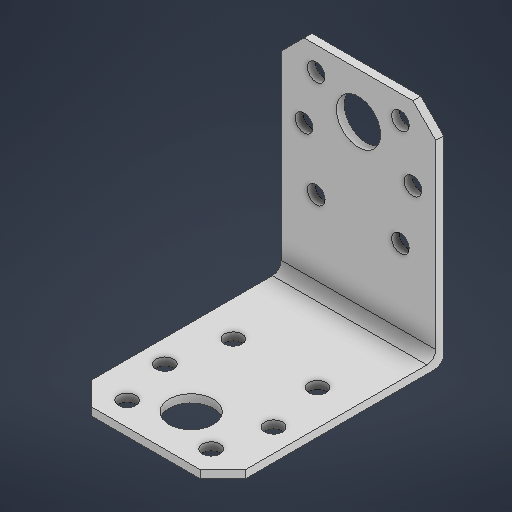
# Autodesk Inventor part: угол для катушки
Saved by Autodesk Inventor 2025 (Build 290162000, 162)
## iProperties
Created: 2025-01-08
Part Number: угол для катушки
Material: Типовые
Document SubType Name: Modeling
Designer: GameHD
Density: 1 g/cm^3
Appearance: По умолчанию
Author: GameHD
Autodesk Inventor part; units mm, degrees
ref_plane "YZ Plane" through (0, 0, 0) normal (1, 0, 0) x (0, 1, 0)
ref_plane "XZ Plane" through (0, 0, 0) normal (0, 1, 0) x (-1, 0, 0)
ref_plane "XY Plane" through (0, 0, 0) normal (0, 0, 1) x (1, 0, 0)
sketch "Эскиз1" plane through (0, 0, 0) normal (0, 0, 1) x (1, 0, 0)
  line L0 (0, 0) -> (35, 0)
  line L1 (35, 0) -> (35, 50)
  line L2 (35, 50) -> (0, 50)
  line L3 (0, 50) -> (0, 0)
  dimension "d0" = 35
  dimension "d1" = 50
  constraints: 8 end point, 2 parallel, 1 horizontal, 1 perpendicular
  measures "d0" distance of L2.end L1.end
  measures "d1" distance of L1.end L0.end
extrude "Выдавливание1" add sketch "Эскиз1" along normal blind 1.8
sketch "Эскиз2" plane through (0, 0, 1.8) normal (0, 0, 1) x (1, 0, 0)
  line L0 (0, 0) -> (35, 0)
  line L1 (35, 0) -> (35, 1.8)
  line L2 (35, 1.8) -> (0, 1.8)
  line L3 (0, 1.8) -> (0, 0)
  dimension "d5" = 35
  dimension "d6" = 1.8
  constraints: 8 end point, 2 parallel, 1 horizontal, 1 perpendicular
  measures "d5" distance of L2.end L1.end
  measures "d6" distance of L1.end L0.end
extrude "Выдавливание2" add sketch "Эскиз2" along normal blind 48.2
fillet "Сопряжение1" radius 2 2 edges at (17.5, 1.8, 1.8) (17.5, 0, 0)
chamfer "Фаска1" distance 5.175 angle 45 4 edges at (0, 50, 0.9) (0, 0.9, 50) (35, 0.9, 50) (35, 50, 0.9)
sketch "Эскиз3" plane through (0, 0, 1.8) normal (0, 0, 1) x (1, 0, 0)
  line L0 (29.825, 50) -> (5.175, 50) projected
  line L1 (17.5, 50) -> (17.5, 1.8)
  line L2 (0, 1.8) -> (35, 1.8) projected
  line L3 (29.825, 50) -> (5.175, 50) projected
  circle A0 centre (17.5, 39.6875) radius 5
  circle A1 centre (7.9375, 44.6875) radius 2
  circle A2 centre (26.9875, 44.6875) radius 2
  circle A3 centre (5.175, 33.3375) radius 2
  circle A4 centre (29.825, 33.3375) radius 2
  circle A5 centre (7.9375, 20.6375) radius 2
  circle A6 centre (26.9875, 20.6375) radius 2
  point P0 (0, 0)
  dimension "d14" = 10
  dimension "d15" = 4
  dimension "d16" = 4
  dimension "d17" = 4
  dimension "d18" = 4
  dimension "d19" = 4
  dimension "d20" = 4
  constraints: 7 centre point, 2 end point, 2 midpoint, 1 perpendicular, 1 point on line
  measures "d14" diameter of A0
  measures "d15" diameter of A1
  measures "d16" diameter of A2
  measures "d17" diameter of A3
  measures "d18" diameter of A4
  measures "d19" diameter of A5
  measures "d20" diameter of A6
extrude "Выдавливание3" cut sketch "Эскиз3" against normal blind 48.2
sketch "Эскиз4" plane through (0, 1.8, 3.8) normal (0, 1, 0) x (1, 0, 0)
  line L0 (5.175, -46.2) -> (29.825, -46.2)
  line L1 (5.175, -46.2) -> (29.825, -46.2)
  circle A0 centre (17.5, -35.8875) radius 5
  circle A1 centre (27.0625, -40.8875) radius 2
  circle A2 centre (8.0125, -40.8875) radius 2
  circle A3 centre (29.825, -29.5375) radius 2
  circle A4 centre (5.175, -29.5375) radius 2
  circle A5 centre (27.0625, -16.8375) radius 2
  circle A6 centre (8.0125, -16.8375) radius 2
  line L2 (29.825, -46.2) -> (5.175, -46.2) projected
  point P0 (0, 3.8)
  point P1 (17.5, -46.2)
  dimension "d23" = 10
  dimension "d24" = 4
  dimension "d25" = 4
  dimension "d26" = 4
  dimension "d27" = 4
  dimension "d28" = 4
  dimension "d29" = 4
  constraints: 7 centre point, 4 end point, 1 coincident, 1 midpoint
  measures "d23" diameter of A0
  measures "d24" diameter of A1
  measures "d25" diameter of A2
  measures "d26" diameter of A3
  measures "d27" diameter of A4
  measures "d28" diameter of A5
  measures "d29" diameter of A6
extrude "Выдавливание4" cut sketch "Эскиз4" against normal blind 48.2
